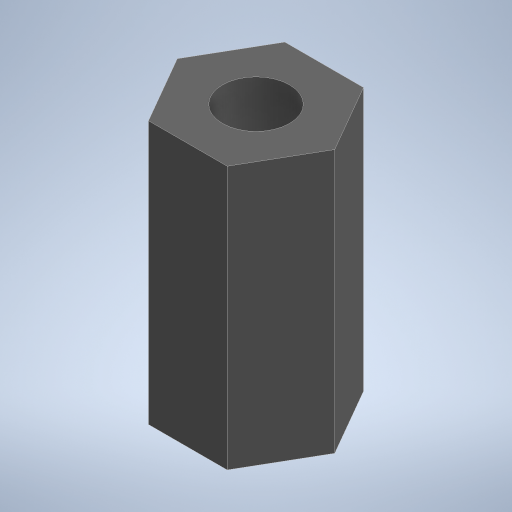
# Autodesk Inventor part: ORCA_board_pole
Saved by Autodesk Inventor 2024.1 (Build 281209000, 209)
## iProperties
Created: 2025-05-30
Part Number: ORCA_board_pole
Material: 一般
Document SubType Name: Modeling
Designer: hibik
Density: 1 g/cm^3
Appearance: 既定
Author: hibik
Autodesk Inventor part; units mm, degrees
ref_plane "YZ Plane" through (0, 0, 0) normal (1, 0, 0) x (0, 1, 0)
ref_plane "XZ Plane" through (0, 0, 0) normal (0, 1, 0) x (-1, 0, 0)
ref_plane "XY Plane" through (0, 0, 0) normal (0, 0, 1) x (1, 0, 0)
sketch "スケッチ1" plane through (0, 0, 0) normal (0, 1, 0) x (-1, 0, 0)
  circle A0 centre (0, 0) radius 1.4
  line L0 (1.6454, -2.85) -> (-1.6454, -2.85)
  line L1 (-1.6454, -2.85) -> (-3.2909, 0)
  line L2 (-3.2909, 0) -> (-1.6454, 2.85)
  line L3 (-1.6454, 2.85) -> (1.6454, 2.85)
  line L4 (1.6454, 2.85) -> (3.2909, 0)
  line L5 (3.2909, 0) -> (1.6454, -2.85)
  dimension "d0" = 2.8
  dimension "d1" = 5.7
  constraints: 12 end point, 2 coincident, 1 centre point, 1 horizontal, 13 other
  measures "d0" diameter of A0
  measures "d1" distance between parallel lines of L2 L5
extrude "押し出し1" add sketch "スケッチ1" along normal blind 11
